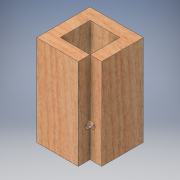
# Autodesk Inventor part: LegHolderOutlet
Saved by Autodesk Inventor 2016 (Build 200138000, 138)
## iProperties
Created: 2016-02-12
Part Number: LegHolderOutlet
Material: Wood (Birch)
Document SubType Name: Modeling
Designer: ron
Density: 0.55 g/cm^3
Appearance: Birch - Natural Polished
Author: ron
Autodesk Inventor part; units mm, degrees
ref_plane "YZ Plane" through (0, 0, 0) normal (1, 0, 0) x (0, 1, 0)
ref_plane "XZ Plane" through (0, 0, 0) normal (0, 1, 0) x (-1, 0, 0)
ref_plane "XY Plane" through (0, 0, 0) normal (0, 0, 1) x (1, 0, 0)
sketch "Sketch1" plane through (0, 0, 0) normal (0, 1, 0) x (-1, 0, 0)
  line L0 (0, 0) -> (20, 0)
  line L1 (20, 0) -> (20, -50.8)
  line L2 (20, -50.8) -> (70.8, -50.8)
  line L3 (70.8, -50.8) -> (70.8, 0)
  line L4 (70.8, 0) -> (20, 0)
  line L5 (0, 0) -> (0, -70.808)
  line L6 (0, -70.808) -> (90.808, -70.808)
  line L7 (90.808, -70.808) -> (90.808, 20.008)
  line L8 (90.808, 20.008) -> (20, 20.008)
  line L9 (20, 20.008) -> (20, 0)
  dimension "d0" = 20
  dimension "d1" = 50.8
  dimension "d2" = 50.8
  dimension "d3" = 50.8
  dimension "d4" = 50.8
  dimension "d6" = 28.2899
  dimension "d7" = 28.2956
  dimension "d8" = 28.2956
  dimension "d11" = 20.008
  constraints: 20 end point, 3 horizontal, 2 parallel, 2 perpendicular, 2 vertical
  measures "d0" distance of L0.start L0.end
  measures "d1" distance of L0.end L1.end
  measures "d2" distance of L1.end L2.end
  measures "d3" distance of L2.end L3.end
  measures "d4" distance of L3.end L0.end
  measures "d6" distance of L1.end L5.end
  measures "d7" distance of L2.end L6.end
  measures "d8" distance of L3.end L7.end
  measures "d11" distance between parallel lines of L3 L7
extrude "Extrusion1" add sketch "Sketch1" along normal blind 155.0924
ref_plane "Work Plane1" through (0, 0, 0) normal (-0.7071068, 0, -0.7071068) x (0, 1, 0)
sketch "Sketch2" plane through (0, 0, 0) normal (-0.7071068, 0, -0.7071068) x (0, 1, 0)
  line L0 (155.0924, 21.7789) -> (155.0924, -14.1421) projected
  line L1 (155.0924, -14.1421) -> (52.705, -14.1421)
  line L2 (0, -14.1421) -> (155.0924, -14.1421) projected
  point P0 (0, 0)
  dimension "d15" = 102.3874
  constraints: 2 end point, 1 point on line
  measures "d15" distance of L0.end L1.end
hole "Hole1" at (-10, 52.705, 10) direction (-0.7071068, 0, -0.7071068) diameter 12.7 depth 25.4
body "Solid1"
